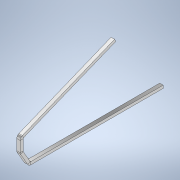
# Autodesk Inventor part: RJ45 Even Pins
Saved by Autodesk Inventor 2020.1 (Build 241239000, 239)
## iProperties
Created: 2019-12-05
Part Number: RJ45 Even Pins
Material: Nickel-Copper Alloy 400
Document SubType Name: Sheet Metal
Designer: S. Lee
Mass: 0.0462409 g
Surface Area: 0.536167 cm^2
Volume: 0.0052368 cm^3
Density: 8.83 g/cm^3
Sheet Metal Rule: Nickel Copper Alloy
Appearance: Chrome - Polished
Author: S. Lee
Autodesk Inventor part; units mm, degrees
ref_plane "YZ Plane" through (0, 0, 0) normal (1, 0, 0) x (0, 1, 0)
ref_plane "XZ Plane" through (0, 0, 0) normal (0, 1, 0) x (-1, 0, 0)
ref_plane "XY Plane" through (0, 0, 0) normal (0, 0, 1) x (1, 0, 0)
sketch "Sketch1" plane through (0, 0, 0) normal (0, 1, 0) x (-1, 0, 0)
  line L0 (0.224, 8.425) -> (-0.224, 8.425)
  line L1 (-0.224, 8.425) -> (-0.224, -8.425)
  line L2 (-0.224, -8.425) -> (0.224, -8.425)
  line L3 (0.224, -8.425) -> (0.224, 8.425)
  line L4 (0.224, 8.425) -> (-0.224, -8.425) construction
  line L5 (-0.224, 8.425) -> (0.224, -8.425) construction
  point P0 (0, 0)
  dimension "d0" = 0.448
  dimension "d1" = 16.85
  measures "d0" distance of L1.end L2.end
  measures "d1" distance of L0.end L1.end
extrude "Plate1" add sketch "Sketch1" along normal blind 0.35
sketch "Sketch2" plane through (0.224, 0.4, 8.5116) normal (0, -0.5, 0.8660254) x (1, 0, 0)
  line L0 (-0.448, 0) -> (0, 0)
  line L1 (0, 0) -> (0, 1.7952)
  line L2 (0, 1.7952) -> (-0.448, 1.7952)
  line L3 (-0.448, 1.7952) -> (-0.448, 0)
  constraints: 6 end point, 1 horizontal, 1 perpendicular, 1 vertical
edge flange "Flange1" height 2.055 angle 60 thickness 0.35 bend radius 0.1 thickness toward (0, -0.5, 0.8660254) relief tear relief width 0.35 relief depth 0.175 edges at (0, 0.35, 8.425) wall of the first edge with corners at (-0.224, 0.4, 8.5116) (0.224, 0.4, 8.5116) (0.224, 1.9547, 9.4092) (-0.224, 1.9547, 9.4092)
bend "Bend1"
corner "Corner1"
sketch "Sketch3" plane through (0.224, 2.0047, 9.4226) normal (0, 0, 1) x (1, 0, 0)
  line L0 (-0.448, 0) -> (0, 0)
  line L1 (0, 0) -> (0, 1.3479)
  line L2 (0, 1.3479) -> (-0.448, 1.3479)
  line L3 (-0.448, 1.3479) -> (-0.448, 0)
  constraints: 6 end point, 1 horizontal, 1 perpendicular, 1 vertical
edge flange "Flange2" height 1.4685 angle 30 thickness 0.35 bend radius 0.1 thickness toward (0, 0, 1) relief tear relief width 0.35 relief depth 0.175 edges at (0, 1.9547, 9.4092) wall of the first edge with corners at (-0.224, 2.0047, 9.4226) (0.224, 2.0047, 9.4226) (0.224, 3.3526, 9.4226) (-0.224, 3.3526, 9.4226)
bend "Bend2"
corner "Corner2"
sketch "Sketch4" plane through (0.224, 3.4453, 9.3601) normal (0, 0.9271839, 0.3746066) x (-1, 0, 0)
  line L0 (0.448, 0) -> (0, 0)
  line L1 (0, 0) -> (0, -12.6465)
  line L2 (0, -12.6465) -> (0.448, -12.6465)
  line L3 (0.448, -12.6465) -> (0.448, 0)
  constraints: 6 end point, 1 horizontal, 1 perpendicular, 1 vertical
edge flange "Flange3" height 12.95 angle 68 thickness 0.35 bend radius 0.1 thickness toward (0, 0.9271839, 0.3746066) relief tear relief width 0.35 relief depth 0.175 edges at (0, 3.3526, 9.4226) wall of the first edge with corners at (-0.224, 3.4453, 9.3601) (0.224, 3.4453, 9.3601) (0.224, 8.1828, -2.3655) (-0.224, 8.1828, -2.3655)
bend "Bend3"
corner "Corner3"
equation "\"d2\" = Thickness"
equation "\"d3\" = BendReliefWidth"
equation "\"d4\" = BendReliefDepth"
equation "\"d5\" = MinimumRemnant"
equation "\"d6\" = TransitionRadius"
equation "\"d9\" = BendRadius"
equation "\"d10\" = CornerReliefSize"
equation "\"d11\" = GapSize"
equation "\"d12\" = JacobiRadiusSize"
equation "\"d13\" = BendReliefWidth"
equation "\"d14\" = BendReliefDepth"
equation "\"d15\" = MinimumRemnant"
equation "\"d16\" = TransitionRadius"
equation "\"d19\" = BendRadius"
equation "\"d20\" = CornerReliefSize"
equation "\"d21\" = GapSize"
equation "\"d22\" = JacobiRadiusSize"
equation "\"d23\" = BendReliefWidth"
equation "\"d24\" = BendReliefDepth"
equation "\"d25\" = MinimumRemnant"
equation "\"d26\" = TransitionRadius"
equation "\"d29\" = BendRadius"
equation "\"d30\" = CornerReliefSize"
equation "\"d31\" = GapSize"
equation "\"d32\" = JacobiRadiusSize"
equation "\"BendReliefWidth\" = Thickness"
equation "\"BendReliefDepth\" = 0.5 * Thickness"
equation "\"CornerReliefSize\" = 4 * Thickness"
equation "\"MinimumRemnant\" = 2 * Thickness"
equation "\"TransitionRadius\" = BendRadius"
equation "\"JacobiRadiusSize\" = BendRadius"
equation "\"GapSize\" = Thickness"
equation "\"Thickness\" = 0.35"
equation "\"BendRadius\" = 0.1"
body "Solid1"
